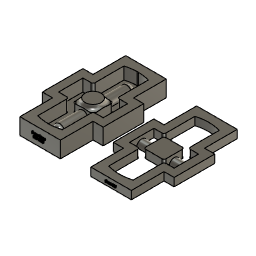
hydrogel_seeding_mould_5mm_diameter v8 (Autodesk Fusion 360 design; units mm, degrees)
Autodesk Fusion 360 part; units mm, degrees
note: some values were not read from the file. Set by a fixed rule: which face or edge a step refers to.
sketch "Sketch1" plane through (0, 0, 0) normal (0, 0, 1) x (1, 0, 0)
  line L0 (5, 13.05) -> (-5, 13.05)
  line L1 (-5, 13.05) -> (-5, -13.05)
  line L2 (-5, -13.05) -> (5, -13.05)
  line L3 (5, -13.05) -> (5, 13.05)
  line L4 (5, 13.05) -> (-5, -13.05) construction
  line L5 (-5, 13.05) -> (5, -13.05) construction
  line L6 (7.5, 5) -> (-7.5, 5)
  line L7 (-7.5, 5) -> (-7.5, -5)
  line L8 (-7.5, -5) -> (7.5, -5)
  line L9 (7.5, -5) -> (7.5, 5)
  line L10 (7.5, 5) -> (-7.5, -5) construction
  line L11 (-7.5, 5) -> (7.5, -5) construction
  dimension "d1" = 10
  dimension "d2" = 26.1
  dimension "d3" = 15
  dimension "d4" = 10
  constraint horizontal L0
  constraint perpendicular L0 L1
  constraint parallel L0 L2
  constraint parallel L1 L3
  constraint coincident L4 origin
  constraint coincident L5 origin
  constraint horizontal L6
  constraint perpendicular L6 L7
  constraint parallel L6 L8
  constraint parallel L7 L9
  constraint coincident L10 origin
  constraint coincident L11 origin
  measures "d1" distance of L1.end L2.end
  measures "d2" distance of L0.end L1.end
  measures "d3" distance of L7.end L8.end
  measures "d4" distance of L6.end L7.end
extrude "Extrude1" add sketch "Sketch1" along normal blind 6 makes body 1
shell "Shell1" thickness 2 removed faces 1 at (1.6667, -1.6667, 6) on bodies 1
extrude "Extrude2" cut 1 faces at (1, -8.3667, 2) along direction (0, 0, -1) blind 1 on bodies 1 bodies 1
sketch "Sketch2" plane through (0, 0, 1) normal (0, 0, 1) x (-1, 0, 0)
  line L0 (-5.5, 3) -> (-5.5, -3)
  line L1 (-5.5, -3) -> (-3, -3)
  line L2 (-3, -3) -> (-3, -11.05)
  line L3 (-3, -11.05) -> (3, -11.05)
  line L4 (3, -11.05) -> (3, -3)
  line L5 (3, -3) -> (5.5, -3)
  line L6 (5.5, -3) -> (5.5, 3)
  line L7 (5.5, 3) -> (3, 3)
  line L8 (3, 3) -> (3, 11.05)
  line L9 (3, 11.05) -> (-3, 11.05)
  line L10 (-3, 11.05) -> (-3, 3)
  line L11 (-3, 3) -> (-5.5, 3)
  line L12 (-2.5, 2.5) -> (2.5, 2.5)
  line L13 (2.5, 2.5) -> (2.5, -2.5)
  line L14 (2.5, -2.5) -> (-2.5, -2.5)
  line L15 (-2.5, -2.5) -> (-2.5, 2.5)
  line L16 (-2.5, 2.5) -> (2.5, -2.5) construction
  line L17 (2.5, 2.5) -> (-2.5, -2.5) construction
  dimension "d10" = 5
  dimension "d11" = 5
  constraint horizontal L12
  constraint perpendicular L12 L13
  constraint parallel L12 L14
  constraint parallel L13 L15
  constraint coincident L16 origin
  constraint coincident L17 origin
  measures "d10" distance of L13.end L14.end
  measures "d11" distance of L12.end L13.end
extrude "Extrude3" add sketch "Sketch2" along normal blind 2 contours L12 L13 L14 L15 bodies 1
sketch "Sketch3" plane through (0, -2.5, 0) normal (0, -1, 0) x (1, 0, 0)
  line L0 (-2.5, 1) -> (2.5, 1)
  line L1 (2.5, 1) -> (2.5, 3)
  line L2 (2.5, 3) -> (-2.5, 3)
  line L3 (-2.5, 3) -> (-2.5, 1)
  circle A0 centre (0, 1.4) radius 1.25
  dimension "d14" = 2.5
  measures "d14" diameter of A0
extrude "Extrude4" add sketch "Sketch3" along normal blind 7 and the other way blind 12 contours L0 A0 picked at (0.3126, 1.4088) bodies 1
fillet "Fillet1" radius 1.25 2 edges at (0, 9.5, 2.65) (0, -9.5, 2.65) on bodies 1
fillet "Fillet2" radius 0.5 4 edges at (-2.5, 2.5, 2) (-2.5, -2.5, 2) (2.5, -2.5, 2) (2.5, 2.5, 2) on bodies 1
fillet "Fillet2" radius 0.5 4 edges at (-3, 3, 3.5) (-3, -3, 3.5) (3, 3, 3.5) (3, -3, 3.5) on bodies 1
sketch "Sketch4" plane through (0, 0, 3) normal (0, 0, 1) x (-1, 0, 0)
  arc A0 (-2.5, -2) -> (-2, -2.5) centre (-2, -2) ccw
  line L0 (-2, -2.5) -> (2, -2.5)
  arc A1 (2, -2.5) -> (2.5, -2) centre (2, -2) ccw
  line L1 (2.5, -2) -> (2.5, 2)
  arc A2 (2.5, 2) -> (2, 2.5) centre (2, 2) ccw
  line L2 (2, 2.5) -> (-2, 2.5)
  arc A3 (-2, 2.5) -> (-2.5, 2) centre (-2, 2) ccw
  line L3 (-2.5, 2) -> (-2.5, -2)
  circle A4 centre (0, 0) radius 2
  constraint coincident A4.centre origin
extrude "Extrude5" add sketch "Sketch4" along normal blind 1 contours A4 bodies 1
sketch "Sketch5" plane through (0, 0, 4) normal (0, 0, 1) x (-1, 0, 0)
  circle A0 centre (0, 0) radius 2
  line L0 (-2.5, -2.5) -> (2.5, -2.5)
  line L1 (2.5, -2.5) -> (2.5, 2.5)
  line L2 (2.5, 2.5) -> (-2.5, 2.5)
  line L3 (-2.5, 2.5) -> (-2.5, -2.5)
  line L4 (-2.5, -2.5) -> (2.5, 2.5) construction
  line L5 (2.5, -2.5) -> (-2.5, 2.5) construction
  dimension "d27" = 5
  dimension "d28" = 5
  constraint horizontal L0
  constraint perpendicular L0 L1
  constraint parallel L0 L2
  constraint parallel L1 L3
  constraint coincident L4 A0.centre
  constraint coincident L5 A0.centre
  constraint coincident A0.centre origin
  measures "d27" distance of L1.end L2.end
  measures "d28" distance of L0.end L1.end
extrude "Extrude6" add sketch "Sketch5" along normal blind 2 contours A0 | L0 L1 L2 L3 bodies 1
fillet "Fillet3" radius 0.5 4 edges at (2.5, -2.5, 5) (-2.5, -2.5, 5) (-2.5, 2.5, 5) (2.5, 2.5, 5) on bodies 1
sketch "Sketch6" plane through (2.5, 0, 0) normal (1, 0, 0) x (0, 1, 0)
  line L0 (2, 4) -> (2, 6)
  line L1 (2, 6) -> (-2, 6)
  line L2 (-2, 6) -> (-2, 4)
  line L3 (-2, 4) -> (2, 4)
  circle A0 centre (0, 6) radius 1.25
  dimension "d33" = 2.5
  constraint midpoint L1 A0.centre
  measures "d33" diameter of A0
extrude "Extrude7" add sketch "Sketch6" along normal blind 3 and the other way blind 8 contours L1 A0 picked at (0.412, 5.4685) bodies 1
fillet "Fillet4" radius 1 1 edges at (1.8647, -0.7232, 3) on bodies 1
sketch "Sketch13" plane through (0, 0, 1) normal (0, 0, 1) x (-1, 0, 0)
  line L0 (1.1843, 8.25) -> (1.1843, 2.5)
  line L1 (1.1843, 2.5) -> (2, 2.5)
  arc A0 (2.5, 2) -> (2, 2.5) centre (2, 2) ccw
  line L2 (2.5, 2) -> (2.5, -2)
  arc A1 (2, -2.5) -> (2.5, -2) centre (2, -2) ccw
  line L3 (2, -2.5) -> (1.1843, -2.5)
  line L4 (1.1843, -2.5) -> (1.1843, -8.25)
  arc A2 (-1.1843, -8.25) -> (1.1843, -8.25) centre (0, -8.25) ccw
  line L5 (-1.1843, -8.25) -> (-1.1843, -2.5)
  line L6 (-1.1843, -2.5) -> (-2, -2.5)
  arc A3 (-2.5, -2) -> (-2, -2.5) centre (-2, -2) ccw
  line L7 (-2.5, -2) -> (-2.5, 2)
  arc A4 (-2, 2.5) -> (-2.5, 2) centre (-2, 2) ccw
  line L8 (-2, 2.5) -> (-1.1843, 2.5)
  line L9 (-1.1843, 2.5) -> (-1.1843, 8.25)
  arc A5 (1.1843, 8.25) -> (-1.1843, 8.25) centre (0, 8.25) ccw
  line L10 (-5.5, 3) -> (-5.5, -3)
  line L11 (-5.5, -3) -> (-3.5, -3)
  arc A6 (-3, -3.5) -> (-3.5, -3) centre (-3.5, -3.5) ccw
  line L12 (-3, -3.5) -> (-3, -11.05)
  line L13 (-3, -11.05) -> (3, -11.05)
  line L14 (3, -11.05) -> (3, -3.5)
  arc A7 (3.5, -3) -> (3, -3.5) centre (3.5, -3.5) ccw
  line L15 (3.5, -3) -> (5.5, -3)
  line L16 (5.5, -3) -> (5.5, 3)
  line L17 (5.5, 3) -> (3.5, 3)
  arc A8 (3, 3.5) -> (3.5, 3) centre (3.5, 3.5) ccw
  line L18 (3, 3.5) -> (3, 11.05)
  line L19 (3, 11.05) -> (-3, 11.05)
  line L20 (-3, 11.05) -> (-3, 3.5)
  arc A9 (-3.5, 3) -> (-3, 3.5) centre (-3.5, 3.5) ccw
  line L21 (-3.5, 3) -> (-5.5, 3)
  arc A10 (-3, -10.5979) -> (3, -10.6142) centre (0.0269, -0.7177) ccw
  arc A11 (3, 10.606) -> (-3, 10.6047) centre (0.0021, 0.6049) ccw
  constraint coincident L12 A10.start
  constraint coincident L14 A10.end
  constraint coincident L18 A11.start
  constraint coincident L20 A11.end
extrude "Extrude8" add sketch "Sketch13" along normal blind 5 contours L18 L19 L20 A11 | L12 L13 A10 | L13 L14 A10 bodies 1
ref_plane "WorkPlane3" through (0, 0, 4) normal (0, 0, -1) x (-1, 0, 0)
split "Split1" by plane through (0, 0, 4) normal (0, 0, -1) bodies 1 makes body 2 at (1.6667, -1.6667, 0)
move_body "Move1" bodies 1 to x (1, 0, 0) y (0, 1, 0) z (0, 0, 1) at (17.5, 0, 0)
move_body "Move2" bodies 1 to x (1, 0, 0) y (0, -1, 0) z (0, 0, -1) at (0, 5, 8)
move_body "Move3" bodies 1 to x (1, 0, 0) y (0, 1, 0) z (0, 0, 1) at (0, 0, -2)
move_body "Move4" bodies 1 to x (1, 0, 0) y (0, 1, 0) z (0, 0, 1) at (0, -5, 0)
sketch "Sketch14" plane through (0, -13.05, 0) normal (0, -1, 0) x (1, 0, 0)
  line L0 (5, 4) -> (-5, 4)
  line L1 (-5, 4) -> (-5, 0)
  line L2 (-5, 0) -> (5, 0)
  line L3 (5, 0) -> (5, 4)
  line L4 (16.2005, 0.881) -> (16.265, 0.8864)
  spline S0 degree 2 poles (16.265, 0.8864) (16.2722, 0.8394) (16.2983, 0.8157) knots 0 0 0 1 1 1
  spline S1 degree 2 poles (16.2983, 0.8157) (16.3244, 0.792) (16.3612, 0.792) knots 0 0 0 1 1 1
  spline S2 degree 2 poles (16.3612, 0.792) (16.4055, 0.792) (16.4362, 0.8254) knots 0 0 0 1 1 1
  spline S3 degree 2 poles (16.4362, 0.8254) (16.4669, 0.8588) (16.4669, 0.9141) knots 0 0 0 1 1 1
  spline S4 degree 2 poles (16.4669, 0.9141) (16.4669, 0.9666) (16.4374, 0.9969) knots 0 0 0 1 1 1
  spline S5 degree 2 poles (16.4374, 0.9969) (16.4079, 1.0273) (16.3602, 1.0273) knots 0 0 0 1 1 1
  spline S6 degree 2 poles (16.3602, 1.0273) (16.3305, 1.0273) (16.3066, 1.0138) knots 0 0 0 1 1 1
  spline S7 degree 2 poles (16.3066, 1.0138) (16.2827, 1.0003) (16.2691, 0.9789) knots 0 0 0 1 1 1
  line L5 (16.2691, 0.9789) -> (16.2115, 0.9864)
  line L6 (16.2115, 0.9864) -> (16.2599, 1.2432)
  line L7 (16.2599, 1.2432) -> (16.5085, 1.2432)
  line L8 (16.5085, 1.2432) -> (16.5085, 1.1845)
  line L9 (16.5085, 1.1845) -> (16.309, 1.1845)
  line L10 (16.309, 1.1845) -> (16.2821, 1.0501)
  spline S8 degree 2 poles (16.2821, 1.0501) (16.3271, 1.0815) (16.3765, 1.0815) knots 0 0 0 1 1 1
  spline S9 degree 2 poles (16.3765, 1.0815) (16.442, 1.0815) (16.487, 1.0362) knots 0 0 0 1 1 1
  spline S10 degree 2 poles (16.487, 1.0362) (16.5321, 0.9908) (16.5321, 0.9195) knots 0 0 0 1 1 1
  spline S11 degree 2 poles (16.5321, 0.9195) (16.5321, 0.8516) (16.4925, 0.8022) knots 0 0 0 1 1 1
  spline S12 degree 2 poles (16.4925, 0.8022) (16.4444, 0.7415) (16.3612, 0.7415) knots 0 0 0 1 1 1
  spline S13 degree 2 poles (16.3612, 0.7415) (16.293, 0.7415) (16.2498, 0.7797) knots 0 0 0 1 1 1
  spline S14 degree 2 poles (16.2498, 0.7797) (16.2067, 0.8179) (16.2005, 0.881) knots 0 0 0 1 1 1
  line L11 (16.6061, 0.75) -> (16.6061, 1.1122)
  line L12 (16.6061, 1.1122) -> (16.661, 1.1122)
  line L13 (16.661, 1.1122) -> (16.661, 1.0614)
  spline S15 degree 2 poles (16.661, 1.0614) (16.678, 1.088) (16.7063, 1.1042) knots 0 0 0 1 1 1
  spline S16 degree 2 poles (16.7063, 1.1042) (16.7347, 1.1204) (16.7708, 1.1204) knots 0 0 0 1 1 1
  spline S17 degree 2 poles (16.7708, 1.1204) (16.8111, 1.1204) (16.8368, 1.1037) knots 0 0 0 1 1 1
  spline S18 degree 2 poles (16.8368, 1.1037) (16.8626, 1.087) (16.8731, 1.057) knots 0 0 0 1 1 1
  spline S19 degree 2 poles (16.8731, 1.057) (16.9161, 1.1204) (16.985, 1.1204) knots 0 0 0 1 1 1
  spline S20 degree 2 poles (16.985, 1.1204) (17.0389, 1.1204) (17.0679, 1.0906) knots 0 0 0 1 1 1
  spline S21 degree 2 poles (17.0679, 1.0906) (17.0969, 1.0607) (17.0969, 0.9986) knots 0 0 0 1 1 1
  line L14 (17.0969, 0.9986) -> (17.0969, 0.75)
  line L15 (17.0969, 0.75) -> (17.0358, 0.75)
  line L16 (17.0358, 0.75) -> (17.0358, 0.9782)
  spline S22 degree 2 poles (17.0358, 0.9782) (17.0358, 1.015) (17.0298, 1.0312) knots 0 0 0 1 1 1
  spline S23 degree 2 poles (17.0298, 1.0312) (17.0239, 1.0474) (17.0082, 1.0573) knots 0 0 0 1 1 1
  spline S24 degree 2 poles (17.0082, 1.0573) (16.9925, 1.0672) (16.9714, 1.0672) knots 0 0 0 1 1 1
  spline S25 degree 2 poles (16.9714, 1.0672) (16.9332, 1.0672) (16.9079, 1.0418) knots 0 0 0 1 1 1
  spline S26 degree 2 poles (16.9079, 1.0418) (16.8827, 1.0164) (16.8827, 0.9604) knots 0 0 0 1 1 1
  line L17 (16.8827, 0.9604) -> (16.8827, 0.75)
  line L18 (16.8827, 0.75) -> (16.8213, 0.75)
  line L19 (16.8213, 0.75) -> (16.8213, 0.9853)
  spline S27 degree 2 poles (16.8213, 0.9853) (16.8213, 1.0263) (16.8063, 1.0467) knots 0 0 0 1 1 1
  spline S28 degree 2 poles (16.8063, 1.0467) (16.7913, 1.0672) (16.7572, 1.0672) knots 0 0 0 1 1 1
  spline S29 degree 2 poles (16.7572, 1.0672) (16.7312, 1.0672) (16.7092, 1.0535) knots 0 0 0 1 1 1
  spline S30 degree 2 poles (16.7092, 1.0535) (16.6872, 1.0399) (16.6774, 1.0136) knots 0 0 0 1 1 1
  spline S31 degree 2 poles (16.6774, 1.0136) (16.6675, 0.9874) (16.6675, 0.9379) knots 0 0 0 1 1 1
  line L20 (16.6675, 0.9379) -> (16.6675, 0.75)
  line L21 (16.6675, 0.75) -> (16.6061, 0.75)
  line L22 (17.1879, 0.75) -> (17.1879, 1.1122)
  line L23 (17.1879, 1.1122) -> (17.2428, 1.1122)
  line L24 (17.2428, 1.1122) -> (17.2428, 1.0614)
  spline S32 degree 2 poles (17.2428, 1.0614) (17.2599, 1.088) (17.2882, 1.1042) knots 0 0 0 1 1 1
  spline S33 degree 2 poles (17.2882, 1.1042) (17.3165, 1.1204) (17.3527, 1.1204) knots 0 0 0 1 1 1
  spline S34 degree 2 poles (17.3527, 1.1204) (17.3929, 1.1204) (17.4187, 1.1037) knots 0 0 0 1 1 1
  spline S35 degree 2 poles (17.4187, 1.1037) (17.4444, 1.087) (17.455, 1.057) knots 0 0 0 1 1 1
  spline S36 degree 2 poles (17.455, 1.057) (17.498, 1.1204) (17.5668, 1.1204) knots 0 0 0 1 1 1
  spline S37 degree 2 poles (17.5668, 1.1204) (17.6207, 1.1204) (17.6497, 1.0906) knots 0 0 0 1 1 1
  spline S38 degree 2 poles (17.6497, 1.0906) (17.6787, 1.0607) (17.6787, 0.9986) knots 0 0 0 1 1 1
  line L25 (17.6787, 0.9986) -> (17.6787, 0.75)
  line L26 (17.6787, 0.75) -> (17.6177, 0.75)
  line L27 (17.6177, 0.75) -> (17.6177, 0.9782)
  spline S39 degree 2 poles (17.6177, 0.9782) (17.6177, 1.015) (17.6117, 1.0312) knots 0 0 0 1 1 1
  spline S40 degree 2 poles (17.6117, 1.0312) (17.6057, 1.0474) (17.59, 1.0573) knots 0 0 0 1 1 1
  spline S41 degree 2 poles (17.59, 1.0573) (17.5744, 1.0672) (17.5532, 1.0672) knots 0 0 0 1 1 1
  spline S42 degree 2 poles (17.5532, 1.0672) (17.515, 1.0672) (17.4898, 1.0418) knots 0 0 0 1 1 1
  spline S43 degree 2 poles (17.4898, 1.0418) (17.4645, 1.0164) (17.4645, 0.9604) knots 0 0 0 1 1 1
  line L28 (17.4645, 0.9604) -> (17.4645, 0.75)
  line L29 (17.4645, 0.75) -> (17.4031, 0.75)
  line L30 (17.4031, 0.75) -> (17.4031, 0.9853)
  spline S44 degree 2 poles (17.4031, 0.9853) (17.4031, 1.0263) (17.3881, 1.0467) knots 0 0 0 1 1 1
  spline S45 degree 2 poles (17.3881, 1.0467) (17.3731, 1.0672) (17.339, 1.0672) knots 0 0 0 1 1 1
  spline S46 degree 2 poles (17.339, 1.0672) (17.3131, 1.0672) (17.2911, 1.0535) knots 0 0 0 1 1 1
  spline S47 degree 2 poles (17.2911, 1.0535) (17.2691, 1.0399) (17.2592, 1.0136) knots 0 0 0 1 1 1
  spline S48 degree 2 poles (17.2592, 1.0136) (17.2493, 0.9874) (17.2493, 0.9379) knots 0 0 0 1 1 1
  line L31 (17.2493, 0.9379) -> (17.2493, 0.75)
  line L32 (17.2493, 0.75) -> (17.1879, 0.75)
  line L33 (17.969, 0.75) -> (17.969, 1.25)
  line L34 (17.969, 1.25) -> (18.0351, 1.25)
  line L35 (18.0351, 1.25) -> (18.0351, 0.809)
  line L36 (18.0351, 0.809) -> (18.2814, 0.809)
  line L37 (18.2814, 0.809) -> (18.2814, 0.75)
  line L38 (18.2814, 0.75) -> (17.969, 0.75)
  line L39 (18.3527, 1.1794) -> (18.3527, 1.25)
  line L40 (18.3527, 1.25) -> (18.4141, 1.25)
  line L41 (18.4141, 1.25) -> (18.4141, 1.1794)
  line L42 (18.4141, 1.1794) -> (18.3527, 1.1794)
  line L43 (18.3527, 0.75) -> (18.3527, 1.1122)
  line L44 (18.3527, 1.1122) -> (18.4141, 1.1122)
  line L45 (18.4141, 1.1122) -> (18.4141, 0.75)
  line L46 (18.4141, 0.75) -> (18.3527, 0.75)
  line L47 (18.7425, 0.75) -> (18.7425, 0.7957)
  spline S49 degree 2 poles (18.7425, 0.7957) (18.708, 0.7418) (18.6412, 0.7418) knots 0 0 0 1 1 1
  spline S50 degree 2 poles (18.6412, 0.7418) (18.5979, 0.7418) (18.5616, 0.7657) knots 0 0 0 1 1 1
  spline S51 degree 2 poles (18.5616, 0.7657) (18.5252, 0.7896) (18.5053, 0.8324) knots 0 0 0 1 1 1
  spline S52 degree 2 poles (18.5053, 0.8324) (18.4853, 0.8752) (18.4853, 0.9308) knots 0 0 0 1 1 1
  spline S53 degree 2 poles (18.4853, 0.9308) (18.4853, 0.985) (18.5034, 1.0292) knots 0 0 0 1 1 1
  spline S54 degree 2 poles (18.5034, 1.0292) (18.5215, 1.0733) (18.5576, 1.0969) knots 0 0 0 1 1 1
  spline S55 degree 2 poles (18.5576, 1.0969) (18.5938, 1.1204) (18.6385, 1.1204) knots 0 0 0 1 1 1
  spline S56 degree 2 poles (18.6385, 1.1204) (18.6712, 1.1204) (18.6968, 1.1066) knots 0 0 0 1 1 1
  spline S57 degree 2 poles (18.6968, 1.1066) (18.7224, 1.0928) (18.7384, 1.0706) knots 0 0 0 1 1 1
  line L48 (18.7384, 1.0706) -> (18.7384, 1.25)
  line L49 (18.7384, 1.25) -> (18.7995, 1.25)
  line L50 (18.7995, 1.25) -> (18.7995, 0.75)
  line L51 (18.7995, 0.75) -> (18.7425, 0.75)
  spline S58 degree 2 poles (18.5484, 0.9308) (18.5484, 0.8612) (18.5778, 0.8267) knots 0 0 0 1 1 1
  spline S59 degree 2 poles (18.5778, 0.8267) (18.6071, 0.7923) (18.647, 0.7923) knots 0 0 0 1 1 1
  spline S60 degree 2 poles (18.647, 0.7923) (18.6872, 0.7923) (18.7154, 0.8252) knots 0 0 0 1 1 1
  spline S61 degree 2 poles (18.7154, 0.8252) (18.7435, 0.8581) (18.7435, 0.9256) knots 0 0 0 1 1 1
  spline S62 degree 2 poles (18.7435, 0.9256) (18.7435, 1) (18.7149, 1.0348) knots 0 0 0 1 1 1
  spline S63 degree 2 poles (18.7149, 1.0348) (18.6862, 1.0696) (18.6443, 1.0696) knots 0 0 0 1 1 1
  spline S64 degree 2 poles (18.6443, 1.0696) (18.6033, 1.0696) (18.5759, 1.0362) knots 0 0 0 1 1 1
  spline S65 degree 2 poles (18.5759, 1.0362) (18.5484, 1.0027) (18.5484, 0.9308) knots 0 0 0 1 1 1
  line L52 (-1.8902, 2.2711) -> (-1.8257, 2.2766)
  spline S66 degree 2 poles (-1.8257, 2.2766) (-1.8186, 2.2295) (-1.7925, 2.2058) knots 0 0 0 1 1 1
  spline S67 degree 2 poles (-1.7925, 2.2058) (-1.7664, 2.1821) (-1.7295, 2.1821) knots 0 0 0 1 1 1
  spline S68 degree 2 poles (-1.7295, 2.1821) (-1.6852, 2.1821) (-1.6545, 2.2156) knots 0 0 0 1 1 1
  spline S69 degree 2 poles (-1.6545, 2.2156) (-1.6238, 2.249) (-1.6238, 2.3042) knots 0 0 0 1 1 1
  spline S70 degree 2 poles (-1.6238, 2.3042) (-1.6238, 2.3568) (-1.6533, 2.3871) knots 0 0 0 1 1 1
  spline S71 degree 2 poles (-1.6533, 2.3871) (-1.6828, 2.4175) (-1.7306, 2.4175) knots 0 0 0 1 1 1
  spline S72 degree 2 poles (-1.7306, 2.4175) (-1.7602, 2.4175) (-1.7841, 2.404) knots 0 0 0 1 1 1
  spline S73 degree 2 poles (-1.7841, 2.404) (-1.808, 2.3905) (-1.8216, 2.369) knots 0 0 0 1 1 1
  line L53 (-1.8216, 2.369) -> (-1.8793, 2.3765)
  line L54 (-1.8793, 2.3765) -> (-1.8308, 2.6334)
  line L55 (-1.8308, 2.6334) -> (-1.5822, 2.6334)
  line L56 (-1.5822, 2.6334) -> (-1.5822, 2.5747)
  line L57 (-1.5822, 2.5747) -> (-1.7817, 2.5747)
  line L58 (-1.7817, 2.5747) -> (-1.8087, 2.4403)
  spline S74 degree 2 poles (-1.8087, 2.4403) (-1.7636, 2.4717) (-1.7142, 2.4717) knots 0 0 0 1 1 1
  spline S75 degree 2 poles (-1.7142, 2.4717) (-1.6487, 2.4717) (-1.6037, 2.4263) knots 0 0 0 1 1 1
  spline S76 degree 2 poles (-1.6037, 2.4263) (-1.5587, 2.381) (-1.5587, 2.3097) knots 0 0 0 1 1 1
  spline S77 degree 2 poles (-1.5587, 2.3097) (-1.5587, 2.2418) (-1.5982, 2.1924) knots 0 0 0 1 1 1
  spline S78 degree 2 poles (-1.5982, 2.1924) (-1.6463, 2.1317) (-1.7295, 2.1317) knots 0 0 0 1 1 1
  spline S79 degree 2 poles (-1.7295, 2.1317) (-1.7977, 2.1317) (-1.8409, 2.1698) knots 0 0 0 1 1 1
  spline S80 degree 2 poles (-1.8409, 2.1698) (-1.884, 2.208) (-1.8902, 2.2711) knots 0 0 0 1 1 1
  line L59 (-1.4847, 2.1402) -> (-1.4847, 2.5024)
  line L60 (-1.4847, 2.5024) -> (-1.4297, 2.5024)
  line L61 (-1.4297, 2.5024) -> (-1.4297, 2.4516)
  spline S81 degree 2 poles (-1.4297, 2.4516) (-1.4127, 2.4782) (-1.3844, 2.4944) knots 0 0 0 1 1 1
  spline S82 degree 2 poles (-1.3844, 2.4944) (-1.3561, 2.5106) (-1.3199, 2.5106) knots 0 0 0 1 1 1
  spline S83 degree 2 poles (-1.3199, 2.5106) (-1.2797, 2.5106) (-1.2539, 2.4939) knots 0 0 0 1 1 1
  spline S84 degree 2 poles (-1.2539, 2.4939) (-1.2282, 2.4771) (-1.2176, 2.4471) knots 0 0 0 1 1 1
  spline S85 degree 2 poles (-1.2176, 2.4471) (-1.1746, 2.5106) (-1.1057, 2.5106) knots 0 0 0 1 1 1
  spline S86 degree 2 poles (-1.1057, 2.5106) (-1.0518, 2.5106) (-1.0229, 2.4807) knots 0 0 0 1 1 1
  spline S87 degree 2 poles (-1.0229, 2.4807) (-0.9939, 2.4509) (-0.9939, 2.3888) knots 0 0 0 1 1 1
  line L62 (-0.9939, 2.3888) -> (-0.9939, 2.1402)
  line L63 (-0.9939, 2.1402) -> (-1.0549, 2.1402)
  line L64 (-1.0549, 2.1402) -> (-1.0549, 2.3683)
  spline S88 degree 2 poles (-1.0549, 2.3683) (-1.0549, 2.4052) (-1.0609, 2.4214) knots 0 0 0 1 1 1
  spline S89 degree 2 poles (-1.0609, 2.4214) (-1.0668, 2.4376) (-1.0825, 2.4475) knots 0 0 0 1 1 1
  spline S90 degree 2 poles (-1.0825, 2.4475) (-1.0982, 2.4574) (-1.1194, 2.4574) knots 0 0 0 1 1 1
  spline S91 degree 2 poles (-1.1194, 2.4574) (-1.1576, 2.4574) (-1.1828, 2.432) knots 0 0 0 1 1 1
  spline S92 degree 2 poles (-1.1828, 2.432) (-1.208, 2.4065) (-1.208, 2.3506) knots 0 0 0 1 1 1
  line L65 (-1.208, 2.3506) -> (-1.208, 2.1402)
  line L66 (-1.208, 2.1402) -> (-1.2694, 2.1402)
  line L67 (-1.2694, 2.1402) -> (-1.2694, 2.3755)
  spline S93 degree 2 poles (-1.2694, 2.3755) (-1.2694, 2.4164) (-1.2844, 2.4369) knots 0 0 0 1 1 1
  spline S94 degree 2 poles (-1.2844, 2.4369) (-1.2995, 2.4574) (-1.3336, 2.4574) knots 0 0 0 1 1 1
  spline S95 degree 2 poles (-1.3336, 2.4574) (-1.3595, 2.4574) (-1.3815, 2.4437) knots 0 0 0 1 1 1
  spline S96 degree 2 poles (-1.3815, 2.4437) (-1.4035, 2.4301) (-1.4134, 2.4038) knots 0 0 0 1 1 1
  spline S97 degree 2 poles (-1.4134, 2.4038) (-1.4233, 2.3776) (-1.4233, 2.3281) knots 0 0 0 1 1 1
  line L68 (-1.4233, 2.3281) -> (-1.4233, 2.1402)
  line L69 (-1.4233, 2.1402) -> (-1.4847, 2.1402)
  line L70 (-0.9028, 2.1402) -> (-0.9028, 2.5024)
  line L71 (-0.9028, 2.5024) -> (-0.8479, 2.5024)
  line L72 (-0.8479, 2.5024) -> (-0.8479, 2.4516)
  spline S98 degree 2 poles (-0.8479, 2.4516) (-0.8308, 2.4782) (-0.8025, 2.4944) knots 0 0 0 1 1 1
  spline S99 degree 2 poles (-0.8025, 2.4944) (-0.7742, 2.5106) (-0.7381, 2.5106) knots 0 0 0 1 1 1
  spline S100 degree 2 poles (-0.7381, 2.5106) (-0.6978, 2.5106) (-0.6721, 2.4939) knots 0 0 0 1 1 1
  spline S101 degree 2 poles (-0.6721, 2.4939) (-0.6463, 2.4771) (-0.6357, 2.4471) knots 0 0 0 1 1 1
  spline S102 degree 2 poles (-0.6357, 2.4471) (-0.5928, 2.5106) (-0.5239, 2.5106) knots 0 0 0 1 1 1
  spline S103 degree 2 poles (-0.5239, 2.5106) (-0.47, 2.5106) (-0.441, 2.4807) knots 0 0 0 1 1 1
  spline S104 degree 2 poles (-0.441, 2.4807) (-0.412, 2.4509) (-0.412, 2.3888) knots 0 0 0 1 1 1
  line L73 (-0.412, 2.3888) -> (-0.412, 2.1402)
  line L74 (-0.412, 2.1402) -> (-0.4731, 2.1402)
  line L75 (-0.4731, 2.1402) -> (-0.4731, 2.3683)
  spline S105 degree 2 poles (-0.4731, 2.3683) (-0.4731, 2.4052) (-0.479, 2.4214) knots 0 0 0 1 1 1
  spline S106 degree 2 poles (-0.479, 2.4214) (-0.485, 2.4376) (-0.5007, 2.4475) knots 0 0 0 1 1 1
  spline S107 degree 2 poles (-0.5007, 2.4475) (-0.5164, 2.4574) (-0.5375, 2.4574) knots 0 0 0 1 1 1
  spline S108 degree 2 poles (-0.5375, 2.4574) (-0.5757, 2.4574) (-0.601, 2.432) knots 0 0 0 1 1 1
  spline S109 degree 2 poles (-0.601, 2.432) (-0.6262, 2.4065) (-0.6262, 2.3506) knots 0 0 0 1 1 1
  line L76 (-0.6262, 2.3506) -> (-0.6262, 2.1402)
  line L77 (-0.6262, 2.1402) -> (-0.6876, 2.1402)
  line L78 (-0.6876, 2.1402) -> (-0.6876, 2.3755)
  spline S110 degree 2 poles (-0.6876, 2.3755) (-0.6876, 2.4164) (-0.7026, 2.4369) knots 0 0 0 1 1 1
  spline S111 degree 2 poles (-0.7026, 2.4369) (-0.7176, 2.4574) (-0.7517, 2.4574) knots 0 0 0 1 1 1
  spline S112 degree 2 poles (-0.7517, 2.4574) (-0.7776, 2.4574) (-0.7996, 2.4437) knots 0 0 0 1 1 1
  spline S113 degree 2 poles (-0.7996, 2.4437) (-0.8216, 2.4301) (-0.8315, 2.4038) knots 0 0 0 1 1 1
  spline S114 degree 2 poles (-0.8315, 2.4038) (-0.8414, 2.3776) (-0.8414, 2.3281) knots 0 0 0 1 1 1
  line L79 (-0.8414, 2.3281) -> (-0.8414, 2.1402)
  line L80 (-0.8414, 2.1402) -> (-0.9028, 2.1402)
  line L81 (-0.1218, 2.1402) -> (-0.1218, 2.6402)
  line L82 (-0.1218, 2.6402) -> (0.0658, 2.6402)
  spline S115 degree 2 poles (0.0658, 2.6402) (0.1231, 2.6402) (0.1577, 2.625) knots 0 0 0 1 1 1
  spline S116 degree 2 poles (0.1577, 2.625) (0.1924, 2.6098) (0.212, 2.5783) knots 0 0 0 1 1 1
  spline S117 degree 2 poles (0.212, 2.5783) (0.2316, 2.5467) (0.2316, 2.5123) knots 0 0 0 1 1 1
  spline S118 degree 2 poles (0.2316, 2.5123) (0.2316, 2.4802) (0.2142, 2.4519) knots 0 0 0 1 1 1
  spline S119 degree 2 poles (0.2142, 2.4519) (0.1968, 2.4236) (0.1617, 2.4062) knots 0 0 0 1 1 1
  spline S120 degree 2 poles (0.1617, 2.4062) (0.207, 2.3929) (0.2314, 2.3608) knots 0 0 0 1 1 1
  spline S121 degree 2 poles (0.2314, 2.3608) (0.2558, 2.3288) (0.2558, 2.2851) knots 0 0 0 1 1 1
  spline S122 degree 2 poles (0.2558, 2.2851) (0.2558, 2.25) (0.241, 2.2198) knots 0 0 0 1 1 1
  spline S123 degree 2 poles (0.241, 2.2198) (0.2261, 2.1896) (0.2043, 2.1733) knots 0 0 0 1 1 1
  spline S124 degree 2 poles (0.2043, 2.1733) (0.1825, 2.1569) (0.1496, 2.1485) knots 0 0 0 1 1 1
  spline S125 degree 2 poles (0.1496, 2.1485) (0.1166, 2.1402) (0.0689, 2.1402) knots 0 0 0 1 1 1
  line L83 (0.0689, 2.1402) -> (-0.1218, 2.1402)
  line L84 (-0.0556, 2.4301) -> (0.0525, 2.4301)
  spline S126 degree 2 poles (0.0525, 2.4301) (0.0965, 2.4301) (0.1156, 2.4359) knots 0 0 0 1 1 1
  spline S127 degree 2 poles (0.1156, 2.4359) (0.1409, 2.4434) (0.1536, 2.4608) knots 0 0 0 1 1 1
  spline S128 degree 2 poles (0.1536, 2.4608) (0.1664, 2.4782) (0.1664, 2.5044) knots 0 0 0 1 1 1
  spline S129 degree 2 poles (0.1664, 2.5044) (0.1664, 2.5293) (0.1545, 2.5483) knots 0 0 0 1 1 1
  spline S130 degree 2 poles (0.1545, 2.5483) (0.1426, 2.5672) (0.1204, 2.5742) knots 0 0 0 1 1 1
  spline S131 degree 2 poles (0.1204, 2.5742) (0.0982, 2.5812) (0.0443, 2.5812) knots 0 0 0 1 1 1
  line L85 (0.0443, 2.5812) -> (-0.0556, 2.5812)
  line L86 (-0.0556, 2.5812) -> (-0.0556, 2.4301)
  line L87 (-0.0556, 2.1992) -> (0.0689, 2.1992)
  spline S132 degree 2 poles (0.0689, 2.1992) (0.101, 2.1992) (0.1139, 2.2016) knots 0 0 0 1 1 1
  spline S133 degree 2 poles (0.1139, 2.2016) (0.1368, 2.2057) (0.1521, 2.2152) knots 0 0 0 1 1 1
  spline S134 degree 2 poles (0.1521, 2.2152) (0.1675, 2.2248) (0.1774, 2.243) knots 0 0 0 1 1 1
  spline S135 degree 2 poles (0.1774, 2.243) (0.1872, 2.2613) (0.1872, 2.2851) knots 0 0 0 1 1 1
  spline S136 degree 2 poles (0.1872, 2.2851) (0.1872, 2.3131) (0.1729, 2.3337) knots 0 0 0 1 1 1
  spline S137 degree 2 poles (0.1729, 2.3337) (0.1586, 2.3544) (0.1332, 2.3627) knots 0 0 0 1 1 1
  spline S138 degree 2 poles (0.1332, 2.3627) (0.1078, 2.3711) (0.06, 2.3711) knots 0 0 0 1 1 1
  line L88 (0.06, 2.3711) -> (-0.0556, 2.3711)
  line L89 (-0.0556, 2.3711) -> (-0.0556, 2.1992)
  spline S139 degree 2 poles (0.5754, 2.1849) (0.5413, 2.1559) (0.5097, 2.1439) knots 0 0 0 1 1 1
  spline S140 degree 2 poles (0.5097, 2.1439) (0.4782, 2.132) (0.442, 2.132) knots 0 0 0 1 1 1
  spline S141 degree 2 poles (0.442, 2.132) (0.3823, 2.132) (0.3503, 2.1612) knots 0 0 0 1 1 1
  spline S142 degree 2 poles (0.3503, 2.1612) (0.3182, 2.1903) (0.3182, 2.2357) knots 0 0 0 1 1 1
  spline S143 degree 2 poles (0.3182, 2.2357) (0.3182, 2.2623) (0.3303, 2.2843) knots 0 0 0 1 1 1
  spline S144 degree 2 poles (0.3303, 2.2843) (0.3424, 2.3063) (0.362, 2.3196) knots 0 0 0 1 1 1
  spline S145 degree 2 poles (0.362, 2.3196) (0.3817, 2.3329) (0.4062, 2.3397) knots 0 0 0 1 1 1
  spline S146 degree 2 poles (0.4062, 2.3397) (0.4243, 2.3445) (0.4608, 2.3489) knots 0 0 0 1 1 1
  spline S147 degree 2 poles (0.4608, 2.3489) (0.5351, 2.3578) (0.5703, 2.3701) knots 0 0 0 1 1 1
  spline S148 degree 2 poles (0.5703, 2.3701) (0.5706, 2.3827) (0.5706, 2.3861) knots 0 0 0 1 1 1
  spline S149 degree 2 poles (0.5706, 2.3861) (0.5706, 2.4236) (0.5532, 2.4389) knots 0 0 0 1 1 1
  spline S150 degree 2 poles (0.5532, 2.4389) (0.5297, 2.4598) (0.4833, 2.4598) knots 0 0 0 1 1 1
  spline S151 degree 2 poles (0.4833, 2.4598) (0.44, 2.4598) (0.4193, 2.4446) knots 0 0 0 1 1 1
  spline S152 degree 2 poles (0.4193, 2.4446) (0.3987, 2.4294) (0.3888, 2.3909) knots 0 0 0 1 1 1
  line L90 (0.3888, 2.3909) -> (0.3288, 2.399)
  spline S153 degree 2 poles (0.3288, 2.399) (0.337, 2.4376) (0.3557, 2.4613) knots 0 0 0 1 1 1
  spline S154 degree 2 poles (0.3557, 2.4613) (0.3745, 2.485) (0.41, 2.4978) knots 0 0 0 1 1 1
  spline S155 degree 2 poles (0.41, 2.4978) (0.4454, 2.5106) (0.4922, 2.5106) knots 0 0 0 1 1 1
  spline S156 degree 2 poles (0.4922, 2.5106) (0.5385, 2.5106) (0.5675, 2.4997) knots 0 0 0 1 1 1
  spline S157 degree 2 poles (0.5675, 2.4997) (0.5965, 2.4887) (0.6102, 2.4722) knots 0 0 0 1 1 1
  spline S158 degree 2 poles (0.6102, 2.4722) (0.6238, 2.4557) (0.6293, 2.4304) knots 0 0 0 1 1 1
  spline S159 degree 2 poles (0.6293, 2.4304) (0.6323, 2.4147) (0.6323, 2.3738) knots 0 0 0 1 1 1
  line L91 (0.6323, 2.3738) -> (0.6323, 2.292)
  spline S160 degree 2 poles (0.6323, 2.292) (0.6323, 2.2063) (0.6363, 2.1837) knots 0 0 0 1 1 1
  spline S161 degree 2 poles (0.6363, 2.1837) (0.6402, 2.161) (0.6518, 2.1402) knots 0 0 0 1 1 1
  line L92 (0.6518, 2.1402) -> (0.5877, 2.1402)
  spline S162 degree 2 poles (0.5877, 2.1402) (0.5781, 2.1593) (0.5754, 2.1849) knots 0 0 0 1 1 1
  spline S163 degree 2 poles (0.5703, 2.322) (0.5368, 2.3083) (0.47, 2.2988) knots 0 0 0 1 1 1
  spline S164 degree 2 poles (0.47, 2.2988) (0.4321, 2.2933) (0.4164, 2.2865) knots 0 0 0 1 1 1
  spline S165 degree 2 poles (0.4164, 2.2865) (0.4008, 2.2797) (0.3922, 2.2665) knots 0 0 0 1 1 1
  spline S166 degree 2 poles (0.3922, 2.2665) (0.3837, 2.2534) (0.3837, 2.2374) knots 0 0 0 1 1 1
  spline S167 degree 2 poles (0.3837, 2.2374) (0.3837, 2.2128) (0.4023, 2.1965) knots 0 0 0 1 1 1
  spline S168 degree 2 poles (0.4023, 2.1965) (0.4209, 2.1801) (0.4567, 2.1801) knots 0 0 0 1 1 1
  spline S169 degree 2 poles (0.4567, 2.1801) (0.4922, 2.1801) (0.5198, 2.1956) knots 0 0 0 1 1 1
  spline S170 degree 2 poles (0.5198, 2.1956) (0.5474, 2.2111) (0.5604, 2.2381) knots 0 0 0 1 1 1
  spline S171 degree 2 poles (0.5604, 2.2381) (0.5703, 2.2589) (0.5703, 2.2995) knots 0 0 0 1 1 1
  line L93 (0.5703, 2.2995) -> (0.5703, 2.322)
  line L94 (0.7029, 2.2483) -> (0.7636, 2.2578)
  spline S172 degree 2 poles (0.7636, 2.2578) (0.7688, 2.2214) (0.7921, 2.2019) knots 0 0 0 1 1 1
  spline S173 degree 2 poles (0.7921, 2.2019) (0.8155, 2.1825) (0.8574, 2.1825) knots 0 0 0 1 1 1
  spline S174 degree 2 poles (0.8574, 2.1825) (0.8997, 2.1825) (0.9202, 2.1997) knots 0 0 0 1 1 1
  spline S175 degree 2 poles (0.9202, 2.1997) (0.9407, 2.2169) (0.9407, 2.2401) knots 0 0 0 1 1 1
  spline S176 degree 2 poles (0.9407, 2.2401) (0.9407, 2.2609) (0.9226, 2.2729) knots 0 0 0 1 1 1
  spline S177 degree 2 poles (0.9226, 2.2729) (0.91, 2.281) (0.8598, 2.2937) knots 0 0 0 1 1 1
  spline S178 degree 2 poles (0.8598, 2.2937) (0.7923, 2.3107) (0.7662, 2.3232) knots 0 0 0 1 1 1
  spline S179 degree 2 poles (0.7662, 2.3232) (0.7401, 2.3356) (0.7266, 2.3576) knots 0 0 0 1 1 1
  spline S180 degree 2 poles (0.7266, 2.3576) (0.7132, 2.3796) (0.7132, 2.4062) knots 0 0 0 1 1 1
  spline S181 degree 2 poles (0.7132, 2.4062) (0.7132, 2.4304) (0.7242, 2.4511) knots 0 0 0 1 1 1
  spline S182 degree 2 poles (0.7242, 2.4511) (0.7353, 2.4717) (0.7544, 2.4853) knots 0 0 0 1 1 1
  spline S183 degree 2 poles (0.7544, 2.4853) (0.7688, 2.4959) (0.7935, 2.5032) knots 0 0 0 1 1 1
  spline S184 degree 2 poles (0.7935, 2.5032) (0.8182, 2.5106) (0.8465, 2.5106) knots 0 0 0 1 1 1
  spline S185 degree 2 poles (0.8465, 2.5106) (0.8892, 2.5106) (0.9214, 2.4983) knots 0 0 0 1 1 1
  spline S186 degree 2 poles (0.9214, 2.4983) (0.9536, 2.486) (0.969, 2.465) knots 0 0 0 1 1 1
  spline S187 degree 2 poles (0.969, 2.465) (0.9843, 2.4441) (0.9901, 2.4089) knots 0 0 0 1 1 1
  line L95 (0.9901, 2.4089) -> (0.9301, 2.4008)
  spline S188 degree 2 poles (0.9301, 2.4008) (0.926, 2.4287) (0.9064, 2.4444) knots 0 0 0 1 1 1
  spline S189 degree 2 poles (0.9064, 2.4444) (0.8868, 2.4601) (0.851, 2.4601) knots 0 0 0 1 1 1
  spline S190 degree 2 poles (0.851, 2.4601) (0.8087, 2.4601) (0.7906, 2.4461) knots 0 0 0 1 1 1
  spline S191 degree 2 poles (0.7906, 2.4461) (0.7725, 2.4321) (0.7725, 2.4134) knots 0 0 0 1 1 1
  spline S192 degree 2 poles (0.7725, 2.4134) (0.7725, 2.4014) (0.78, 2.3919) knots 0 0 0 1 1 1
  spline S193 degree 2 poles (0.78, 2.3919) (0.7875, 2.382) (0.8035, 2.3755) knots 0 0 0 1 1 1
  spline S194 degree 2 poles (0.8035, 2.3755) (0.8128, 2.3721) (0.8578, 2.3598) knots 0 0 0 1 1 1
  spline S195 degree 2 poles (0.8578, 2.3598) (0.9229, 2.3424) (0.9487, 2.3313) knots 0 0 0 1 1 1
  spline S196 degree 2 poles (0.9487, 2.3313) (0.9744, 2.3203) (0.9891, 2.2991) knots 0 0 0 1 1 1
  spline S197 degree 2 poles (0.9891, 2.2991) (1.0038, 2.278) (1.0038, 2.2466) knots 0 0 0 1 1 1
  spline S198 degree 2 poles (1.0038, 2.2466) (1.0038, 2.2159) (0.9858, 2.1888) knots 0 0 0 1 1 1
  spline S199 degree 2 poles (0.9858, 2.1888) (0.9679, 2.1617) (0.9342, 2.1468) knots 0 0 0 1 1 1
  spline S200 degree 2 poles (0.9342, 2.1468) (0.9004, 2.132) (0.8578, 2.132) knots 0 0 0 1 1 1
  spline S201 degree 2 poles (0.8578, 2.132) (0.7872, 2.132) (0.7502, 2.1613) knots 0 0 0 1 1 1
  spline S202 degree 2 poles (0.7502, 2.1613) (0.7132, 2.1907) (0.7029, 2.2483) knots 0 0 0 1 1 1
  line L96 (1.3247, 2.2568) -> (1.3881, 2.249)
  spline S203 degree 2 poles (1.3881, 2.249) (1.3731, 2.1934) (1.3325, 2.1627) knots 0 0 0 1 1 1
  spline S204 degree 2 poles (1.3325, 2.1627) (1.292, 2.132) (1.2289, 2.132) knots 0 0 0 1 1 1
  spline S205 degree 2 poles (1.2289, 2.132) (1.1494, 2.132) (1.1028, 2.1809) knots 0 0 0 1 1 1
  spline S206 degree 2 poles (1.1028, 2.1809) (1.0563, 2.2299) (1.0563, 2.3182) knots 0 0 0 1 1 1
  spline S207 degree 2 poles (1.0563, 2.3182) (1.0563, 2.4096) (1.1033, 2.4601) knots 0 0 0 1 1 1
  spline S208 degree 2 poles (1.1033, 2.4601) (1.1504, 2.5106) (1.2254, 2.5106) knots 0 0 0 1 1 1
  spline S209 degree 2 poles (1.2254, 2.5106) (1.2981, 2.5106) (1.3441, 2.4611) knots 0 0 0 1 1 1
  spline S210 degree 2 poles (1.3441, 2.4611) (1.3902, 2.4117) (1.3902, 2.322) knots 0 0 0 1 1 1
  spline S211 degree 2 poles (1.3902, 2.322) (1.3902, 2.3165) (1.3898, 2.3056) knots 0 0 0 1 1 1
  line L97 (1.3898, 2.3056) -> (1.1197, 2.3056)
  spline S212 degree 2 poles (1.1197, 2.3056) (1.1231, 2.2459) (1.1535, 2.2142) knots 0 0 0 1 1 1
  spline S213 degree 2 poles (1.1535, 2.2142) (1.1838, 2.1825) (1.2292, 2.1825) knots 0 0 0 1 1 1
  spline S214 degree 2 poles (1.2292, 2.1825) (1.263, 2.1825) (1.2868, 2.2002) knots 0 0 0 1 1 1
  spline S215 degree 2 poles (1.2868, 2.2002) (1.3107, 2.2179) (1.3247, 2.2568) knots 0 0 0 1 1 1
  line L98 (1.1231, 2.3561) -> (1.3254, 2.3561)
  spline S216 degree 2 poles (1.3254, 2.3561) (1.3213, 2.4018) (1.3022, 2.4246) knots 0 0 0 1 1 1
  spline S217 degree 2 poles (1.3022, 2.4246) (1.2729, 2.4601) (1.2261, 2.4601) knots 0 0 0 1 1 1
  spline S218 degree 2 poles (1.2261, 2.4601) (1.1838, 2.4601) (1.155, 2.4318) knots 0 0 0 1 1 1
  spline S219 degree 2 poles (1.155, 2.4318) (1.1262, 2.4035) (1.1231, 2.3561) knots 0 0 0 1 1 1
  line L99 (-1.4988, 1.3598) -> (-1.4988, 1.8598)
  line L100 (-1.4988, 1.8598) -> (-1.3992, 1.8598)
  line L101 (-1.3992, 1.8598) -> (-1.2809, 1.5058)
  spline S220 degree 2 poles (-1.2809, 1.5058) (-1.2645, 1.4563) (-1.257, 1.4318) knots 0 0 0 1 1 1
  spline S221 degree 2 poles (-1.257, 1.4318) (-1.2485, 1.4591) (-1.2304, 1.5119) knots 0 0 0 1 1 1
  line L102 (-1.2304, 1.5119) -> (-1.1107, 1.8598)
  line L103 (-1.1107, 1.8598) -> (-1.0217, 1.8598)
  line L104 (-1.0217, 1.8598) -> (-1.0217, 1.3598)
  line L105 (-1.0217, 1.3598) -> (-1.0854, 1.3598)
  line L106 (-1.0854, 1.3598) -> (-1.0854, 1.7783)
  line L107 (-1.0854, 1.7783) -> (-1.2307, 1.3598)
  line L108 (-1.2307, 1.3598) -> (-1.2904, 1.3598)
  line L109 (-1.2904, 1.3598) -> (-1.435, 1.7855)
  line L110 (-1.435, 1.7855) -> (-1.435, 1.3598)
  line L111 (-1.435, 1.3598) -> (-1.4988, 1.3598)
  line L112 (-0.9176, 1.3598) -> (-0.9176, 1.8598)
  line L113 (-0.9176, 1.8598) -> (-0.73, 1.8598)
  spline S222 degree 2 poles (-0.73, 1.8598) (-0.6727, 1.8598) (-0.6381, 1.8446) knots 0 0 0 1 1 1
  spline S223 degree 2 poles (-0.6381, 1.8446) (-0.6035, 1.8295) (-0.5839, 1.7979) knots 0 0 0 1 1 1
  spline S224 degree 2 poles (-0.5839, 1.7979) (-0.5643, 1.7664) (-0.5643, 1.7319) knots 0 0 0 1 1 1
  spline S225 degree 2 poles (-0.5643, 1.7319) (-0.5643, 1.6999) (-0.5817, 1.6716) knots 0 0 0 1 1 1
  spline S226 degree 2 poles (-0.5817, 1.6716) (-0.5991, 1.6432) (-0.6342, 1.6259) knots 0 0 0 1 1 1
  spline S227 degree 2 poles (-0.6342, 1.6259) (-0.5888, 1.6126) (-0.5645, 1.5805) knots 0 0 0 1 1 1
  spline S228 degree 2 poles (-0.5645, 1.5805) (-0.5401, 1.5484) (-0.5401, 1.5048) knots 0 0 0 1 1 1
  spline S229 degree 2 poles (-0.5401, 1.5048) (-0.5401, 1.4696) (-0.5549, 1.4395) knots 0 0 0 1 1 1
  spline S230 degree 2 poles (-0.5549, 1.4395) (-0.5697, 1.4093) (-0.5916, 1.3929) knots 0 0 0 1 1 1
  spline S231 degree 2 poles (-0.5916, 1.3929) (-0.6134, 1.3765) (-0.6463, 1.3682) knots 0 0 0 1 1 1
  spline S232 degree 2 poles (-0.6463, 1.3682) (-0.6792, 1.3598) (-0.727, 1.3598) knots 0 0 0 1 1 1
  line L114 (-0.727, 1.3598) -> (-0.9176, 1.3598)
  line L115 (-0.8515, 1.6497) -> (-0.7433, 1.6497)
  spline S233 degree 2 poles (-0.7433, 1.6497) (-0.6994, 1.6497) (-0.6803, 1.6555) knots 0 0 0 1 1 1
  spline S234 degree 2 poles (-0.6803, 1.6555) (-0.655, 1.663) (-0.6422, 1.6804) knots 0 0 0 1 1 1
  spline S235 degree 2 poles (-0.6422, 1.6804) (-0.6294, 1.6978) (-0.6294, 1.7241) knots 0 0 0 1 1 1
  spline S236 degree 2 poles (-0.6294, 1.7241) (-0.6294, 1.749) (-0.6414, 1.7679) knots 0 0 0 1 1 1
  spline S237 degree 2 poles (-0.6414, 1.7679) (-0.6533, 1.7868) (-0.6755, 1.7938) knots 0 0 0 1 1 1
  spline S238 degree 2 poles (-0.6755, 1.7938) (-0.6976, 1.8008) (-0.7515, 1.8008) knots 0 0 0 1 1 1
  line L116 (-0.7515, 1.8008) -> (-0.8515, 1.8008)
  line L117 (-0.8515, 1.8008) -> (-0.8515, 1.6497)
  line L118 (-0.8515, 1.4188) -> (-0.727, 1.4188)
  spline S239 degree 2 poles (-0.727, 1.4188) (-0.6949, 1.4188) (-0.682, 1.4212) knots 0 0 0 1 1 1
  spline S240 degree 2 poles (-0.682, 1.4212) (-0.6591, 1.4253) (-0.6438, 1.4349) knots 0 0 0 1 1 1
  spline S241 degree 2 poles (-0.6438, 1.4349) (-0.6284, 1.4444) (-0.6185, 1.4627) knots 0 0 0 1 1 1
  spline S242 degree 2 poles (-0.6185, 1.4627) (-0.6086, 1.4809) (-0.6086, 1.5048) knots 0 0 0 1 1 1
  spline S243 degree 2 poles (-0.6086, 1.5048) (-0.6086, 1.5327) (-0.623, 1.5534) knots 0 0 0 1 1 1
  spline S244 degree 2 poles (-0.623, 1.5534) (-0.6373, 1.574) (-0.6627, 1.5824) knots 0 0 0 1 1 1
  spline S245 degree 2 poles (-0.6627, 1.5824) (-0.6881, 1.5907) (-0.7358, 1.5907) knots 0 0 0 1 1 1
  line L119 (-0.7358, 1.5907) -> (-0.8515, 1.5907)
  line L120 (-0.8515, 1.5907) -> (-0.8515, 1.4188)
  line L121 (0.0387, 1.7374) -> (-0.0223, 1.7326)
  spline S246 degree 2 poles (-0.0223, 1.7326) (-0.0305, 1.7688) (-0.0455, 1.7851) knots 0 0 0 1 1 1
  spline S247 degree 2 poles (-0.0455, 1.7851) (-0.0704, 1.8114) (-0.1069, 1.8114) knots 0 0 0 1 1 1
  spline S248 degree 2 poles (-0.1069, 1.8114) (-0.1363, 1.8114) (-0.1584, 1.795) knots 0 0 0 1 1 1
  spline S249 degree 2 poles (-0.1584, 1.795) (-0.1874, 1.7739) (-0.2041, 1.7333) knots 0 0 0 1 1 1
  spline S250 degree 2 poles (-0.2041, 1.7333) (-0.2208, 1.6927) (-0.2215, 1.6177) knots 0 0 0 1 1 1
  spline S251 degree 2 poles (-0.2215, 1.6177) (-0.1994, 1.6514) (-0.1673, 1.6678) knots 0 0 0 1 1 1
  spline S252 degree 2 poles (-0.1673, 1.6678) (-0.1352, 1.6842) (-0.1001, 1.6842) knots 0 0 0 1 1 1
  spline S253 degree 2 poles (-0.1001, 1.6842) (-0.0387, 1.6842) (0.0044, 1.639) knots 0 0 0 1 1 1
  spline S254 degree 2 poles (0.0044, 1.639) (0.0476, 1.5938) (0.0476, 1.5222) knots 0 0 0 1 1 1
  spline S255 degree 2 poles (0.0476, 1.5222) (0.0476, 1.4751) (0.0273, 1.4347) knots 0 0 0 1 1 1
  spline S256 degree 2 poles (0.0273, 1.4347) (0.007, 1.3943) (-0.0285, 1.3728) knots 0 0 0 1 1 1
  spline S257 degree 2 poles (-0.0285, 1.3728) (-0.0639, 1.3513) (-0.109, 1.3513) knots 0 0 0 1 1 1
  spline S258 degree 2 poles (-0.109, 1.3513) (-0.1857, 1.3513) (-0.2341, 1.4077) knots 0 0 0 1 1 1
  spline S259 degree 2 poles (-0.2341, 1.4077) (-0.2826, 1.4642) (-0.2826, 1.5938) knots 0 0 0 1 1 1
  spline S260 degree 2 poles (-0.2826, 1.5938) (-0.2826, 1.7387) (-0.229, 1.8046) knots 0 0 0 1 1 1
  spline S261 degree 2 poles (-0.229, 1.8046) (-0.1823, 1.8619) (-0.1032, 1.8619) knots 0 0 0 1 1 1
  spline S262 degree 2 poles (-0.1032, 1.8619) (-0.0442, 1.8619) (-0.0065, 1.8288) knots 0 0 0 1 1 1
  spline S263 degree 2 poles (-0.0065, 1.8288) (0.0312, 1.7957) (0.0387, 1.7374) knots 0 0 0 1 1 1
  spline S264 degree 2 poles (-0.212, 1.5218) (-0.212, 1.4901) (-0.1985, 1.4611) knots 0 0 0 1 1 1
  spline S265 degree 2 poles (-0.1985, 1.4611) (-0.185, 1.4321) (-0.1608, 1.417) knots 0 0 0 1 1 1
  spline S266 degree 2 poles (-0.1608, 1.417) (-0.1366, 1.4018) (-0.11, 1.4018) knots 0 0 0 1 1 1
  spline S267 degree 2 poles (-0.11, 1.4018) (-0.0711, 1.4018) (-0.0431, 1.4332) knots 0 0 0 1 1 1
  spline S268 degree 2 poles (-0.0431, 1.4332) (-0.0152, 1.4645) (-0.0152, 1.5184) knots 0 0 0 1 1 1
  spline S269 degree 2 poles (-0.0152, 1.5184) (-0.0152, 1.5703) (-0.0428, 1.6001) knots 0 0 0 1 1 1
  spline S270 degree 2 poles (-0.0428, 1.6001) (-0.0704, 1.6299) (-0.1124, 1.6299) knots 0 0 0 1 1 1
  spline S271 degree 2 poles (-0.1124, 1.6299) (-0.154, 1.6299) (-0.183, 1.6001) knots 0 0 0 1 1 1
  spline S272 degree 2 poles (-0.183, 1.6001) (-0.212, 1.5703) (-0.212, 1.5218) knots 0 0 0 1 1 1
  line L122 (0.0796, 1.3513) -> (0.2246, 1.8683)
  line L123 (0.2246, 1.8683) -> (0.2737, 1.8683)
  line L124 (0.2737, 1.8683) -> (0.1291, 1.3513)
  line L125 (0.1291, 1.3513) -> (0.0796, 1.3513)
  line L126 (0.6253, 1.4188) -> (0.6253, 1.3598)
  line L127 (0.6253, 1.3598) -> (0.2949, 1.3598)
  spline S273 degree 2 poles (0.2949, 1.3598) (0.2942, 1.382) (0.302, 1.4025) knots 0 0 0 1 1 1
  spline S274 degree 2 poles (0.302, 1.4025) (0.3146, 1.4362) (0.3424, 1.469) knots 0 0 0 1 1 1
  spline S275 degree 2 poles (0.3424, 1.469) (0.3702, 1.5017) (0.4227, 1.5447) knots 0 0 0 1 1 1
  spline S276 degree 2 poles (0.4227, 1.5447) (0.5043, 1.6115) (0.5329, 1.6506) knots 0 0 0 1 1 1
  spline S277 degree 2 poles (0.5329, 1.6506) (0.5616, 1.6896) (0.5616, 1.7244) knots 0 0 0 1 1 1
  spline S278 degree 2 poles (0.5616, 1.7244) (0.5616, 1.7609) (0.5355, 1.786) knots 0 0 0 1 1 1
  spline S279 degree 2 poles (0.5355, 1.786) (0.5094, 1.8111) (0.4674, 1.8111) knots 0 0 0 1 1 1
  spline S280 degree 2 poles (0.4674, 1.8111) (0.4231, 1.8111) (0.3965, 1.7844) knots 0 0 0 1 1 1
  spline S281 degree 2 poles (0.3965, 1.7844) (0.3699, 1.7578) (0.3695, 1.7108) knots 0 0 0 1 1 1
  line L128 (0.3695, 1.7108) -> (0.3064, 1.7173)
  spline S282 degree 2 poles (0.3064, 1.7173) (0.3129, 1.7879) (0.3552, 1.8249) knots 0 0 0 1 1 1
  spline S283 degree 2 poles (0.3552, 1.8249) (0.3975, 1.8619) (0.4688, 1.8619) knots 0 0 0 1 1 1
  spline S284 degree 2 poles (0.4688, 1.8619) (0.5408, 1.8619) (0.5827, 1.822) knots 0 0 0 1 1 1
  spline S285 degree 2 poles (0.5827, 1.822) (0.6247, 1.7821) (0.6247, 1.7231) knots 0 0 0 1 1 1
  spline S286 degree 2 poles (0.6247, 1.7231) (0.6247, 1.693) (0.6124, 1.6641) knots 0 0 0 1 1 1
  spline S287 degree 2 poles (0.6124, 1.6641) (0.6001, 1.6351) (0.5716, 1.603) knots 0 0 0 1 1 1
  spline S288 degree 2 poles (0.5716, 1.603) (0.5431, 1.5709) (0.477, 1.515) knots 0 0 0 1 1 1
  spline S289 degree 2 poles (0.477, 1.515) (0.4217, 1.4686) (0.406, 1.4521) knots 0 0 0 1 1 1
  spline S290 degree 2 poles (0.406, 1.4521) (0.3903, 1.4355) (0.3801, 1.4188) knots 0 0 0 1 1 1
  line L129 (0.3801, 1.4188) -> (0.6253, 1.4188)
  line L130 (1.0138, 1.4188) -> (1.0138, 1.3598)
  line L131 (1.0138, 1.3598) -> (0.6833, 1.3598)
  spline S291 degree 2 poles (0.6833, 1.3598) (0.6826, 1.382) (0.6905, 1.4025) knots 0 0 0 1 1 1
  spline S292 degree 2 poles (0.6905, 1.4025) (0.7031, 1.4362) (0.7309, 1.469) knots 0 0 0 1 1 1
  spline S293 degree 2 poles (0.7309, 1.469) (0.7587, 1.5017) (0.8112, 1.5447) knots 0 0 0 1 1 1
  spline S294 degree 2 poles (0.8112, 1.5447) (0.8927, 1.6115) (0.9214, 1.6506) knots 0 0 0 1 1 1
  spline S295 degree 2 poles (0.9214, 1.6506) (0.95, 1.6896) (0.95, 1.7244) knots 0 0 0 1 1 1
  spline S296 degree 2 poles (0.95, 1.7244) (0.95, 1.7609) (0.9239, 1.786) knots 0 0 0 1 1 1
  spline S297 degree 2 poles (0.9239, 1.786) (0.8979, 1.8111) (0.8559, 1.8111) knots 0 0 0 1 1 1
  spline S298 degree 2 poles (0.8559, 1.8111) (0.8116, 1.8111) (0.785, 1.7844) knots 0 0 0 1 1 1
  spline S299 degree 2 poles (0.785, 1.7844) (0.7584, 1.7578) (0.758, 1.7108) knots 0 0 0 1 1 1
  line L132 (0.758, 1.7108) -> (0.6949, 1.7173)
  spline S300 degree 2 poles (0.6949, 1.7173) (0.7014, 1.7879) (0.7437, 1.8249) knots 0 0 0 1 1 1
  spline S301 degree 2 poles (0.7437, 1.8249) (0.786, 1.8619) (0.8573, 1.8619) knots 0 0 0 1 1 1
  spline S302 degree 2 poles (0.8573, 1.8619) (0.9292, 1.8619) (0.9712, 1.822) knots 0 0 0 1 1 1
  spline S303 degree 2 poles (0.9712, 1.822) (1.0131, 1.7821) (1.0131, 1.7231) knots 0 0 0 1 1 1
  spline S304 degree 2 poles (1.0131, 1.7231) (1.0131, 1.693) (1.0009, 1.6641) knots 0 0 0 1 1 1
  spline S305 degree 2 poles (1.0009, 1.6641) (0.9886, 1.6351) (0.9601, 1.603) knots 0 0 0 1 1 1
  spline S306 degree 2 poles (0.9601, 1.603) (0.9316, 1.5709) (0.8655, 1.515) knots 0 0 0 1 1 1
  spline S307 degree 2 poles (0.8655, 1.515) (0.8102, 1.4686) (0.7945, 1.4521) knots 0 0 0 1 1 1
  spline S308 degree 2 poles (0.7945, 1.4521) (0.7788, 1.4355) (0.7686, 1.4188) knots 0 0 0 1 1 1
  line L133 (0.7686, 1.4188) -> (1.0138, 1.4188)
extrude "Extrude9" add sketch "Sketch14" along normal blind 0.25 contours L4 S0 S1 S2 S3 S4 S5 S6 S7 L5 L6 L7 L8 L9 L10 S8 S9 S10 S11 S12 S13 S14 | L11 L12 L13 S15 S16 S17 S18 S19 S20 S21 L14 L15 L16 S22 S23 S24 S25 S26 L17 L18 L19 S27 S28 S29 S30 S31 L20 L21 | L22 L23 L24 S32 S33 S34 S35 S36 S37 S38 L25 L26 L27 S39 S40 S41 S42 S43 L28 L29 L30 S44 S45 S46 S47 S48 L31 L32 | L33 L34 L35 L36 L37 L38 | L39 L40 L41 L42 | L43 L44 L45 L46 | L47 S49 S50 S51 S52 S53 S54 S55 S56 S57 L48 L49 L50 L51 | L52 S66 S67 S68 S69 S70 S71 S72 S73 L53 L54 L55 L56 L57 L58 S74 S75 S76 S77 S78 S79 S80 | L59 L60 L61 S81 S82 S83 S84 S85 S86 S87 L62 L63 L64 S88 S89 S90 S91 S92 L65 L66 L67 S93 S94 S95 S96 S97 L68 L69 | L70 L71 L72 S98 S99 S100 S101 S102 S103 S104 L73 L74 L75 S105 S106 S107 S108 S109 L76 L77 L78 S110 S111 S112 S113 S114 L79 L80 | L81 L82 S115 S116 S117 S118 S119 S120 S121 S122 S123 S124 S125 L83 | S139 S140 S141 S142 S143 S144 S145 S146 S147 S148 S149 S150 S151 S152 L90 S153 S154 S155 S156 S157 S158 S159 L91 S160 S161 L92 S162 | L94 S172 S173 S174 S175 S176 S177 S178 S179 S180 S181 S182 S183 S184 S185 S186 S187 L95 S188 S189 S190 S191 S192 S193 S194 S195 S196 S197 S198 S199 S200 S201 S202 | L96 S203 S204 S205 S206 S207 S208 S209 S210 S211 L97 S212 S213 S214 S215 | L99 L100 L101 S220 S221 L102 L103 L104 L105 L106 L107 L108 L109 L110 L111 | L112 L113 S222 S223 S224 S225 S226 S227 S228 S229 S230 S231 S232 L114 | L121 S246 S247 S248 S249 S250 S251 S252 S253 S254 S255 S256 S257 S258 S259 S260 S261 S262 S263 | L122 L123 L124 L125 | L126 L127 S273 S274 S275 S276 S277 S278 S279 S280 S281 L128 S282 S283 S284 S285 S286 S287 S288 S289 S290 L129 | L130 L131 S291 S292 S293 S294 S295 S296 S297 S298 S299 L132 S300 S301 S302 S303 S304 S305 S306 S307 S308 L133 bodies 1 2
